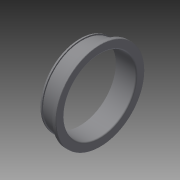
# Autodesk Inventor part: 32912_ir
Saved by Autodesk Inventor 2014 SP2 (Build 180246200, 246)
## iProperties
Created: 2018-11-12
Part Number: 32912_ir
Material: Generic
Catalog Web Link: www.cadenas.de
Description: BT1_001_101_ir-Tapered roller bearings, single row
Vendor: SKF
Document SubType Name: Modeling
Designer: psadmin
Manufacturer: SKF
Mass: 14.0656 g
Surface Area: 94.7996 cm^2
Volume: 14.0656 cm^3
Density: 1 g/cm^3
Appearance: PSOLRGB-175-175-175
Category: PARTsolutions
Company: SKF
Title: 32912_ir
Author: Cadenas PARTsolutions
Comments: Tapered roller bearings, single row
PSOL_IDENT_0: {$CADENAS_DATA\23d-libs\skf\bearings_units_and_housings\roller_bearings\tapered_roller_bearings\tape
PSOL_IDENT_1: red_roller_bearings_single_row\parts\bt1_001_101_ir.prj},166 {VTYP=3D},{NB=32912_ir},{LINA=32912_ir}
PSOL_IDENT_2: ,{NN=BT1_001_101_ir},{DATE=14.08.2018 07:35:10},{GEOMDATE=29.05.2018 10:14:25},{VERSION=},{LINEID=21
PSOL_IDENT_3: 40},{WBVAR=},{WBNUMERIC=}  {NB=32912_ir},{LINA=32912_ir},{KT=DUMMY},{DESIGNATION=32912},{DD=60.000},
PSOL_IDENT_4: {D=85.000},{T=17.000},{DD1=73.8000},{D1=MIN},{B=17.000},{C=14.000},{C1=MIN},{R12=1.0},{R34=1.0},{AA=
PSOL_IDENT_5: 15.45165},{PITCH=72.347},{DW=5.200},{LW=12.200},{RANGLE=1.600},{ALPHA=12.450},{DDAMAX=67},{DDAMIN=68
PSOL_IDENT_6: .0},{DAMIN=78},{DAMAX=78.0},{DBMIN=81},{CA=3},{CB=3.0},{RA=1.0},{RB=1.0},{LOAD1=53.200},{LOAD2=75.00
PSOL_IDENT_7: 0},{LOAD3=7.800},{SPEED1=6000},{SPEED2=7000},{EE=0.33},{Y=1.80},{Y0=1.0},{Y1=0},{X1=1},{X2=0.4},{X0=
PSOL_IDENT_8: 0.5},{Z=34},{II=1},{R1=0.00000231},{R2=10.9},{S1=0.009},{S2=2},{KZ=6},{KL=0.7},{BF=2},{MASS=0.302},{
PSOL_IDENT_9: PIM=PIM_BT1_001},{DESIGN=trb1},{HELP=0.000}
NN: BT1_001_101_ir
NT: Tapered roller bearings, single row
NB: 32912_ir
NBSYN: $DESIGNATION._ir
LINA: 32912_ir
DESIGNATION: 32912
DD: 60
D: 85
T: 17
DD1: 73.8
D1: 0
B: 17
C: 14
C1: 0
R12: 1
R34: 1
AA: 15.45165
PITCH: 72.347
DW: 5.2
LW: 12.2
RANGLE: 1.6
ALPHA: 12.45
DDAMAX: 67
DDAMIN: 68
DAMIN: 78
DAMAX: 78
DBMIN: 81
CA: 3
CB: 3
RA: 1
RB: 1
LOAD1: 53.2
LOAD2: 75
LOAD3: 7.8
SPEED1: 6000
SPEED2: 7000
EE: 0.33
Y: 1.8
Y0: 1
Y1: 0
X1: 1
X2: 0.4
X0: 0.5
Z: 34
II: 1
R1: 0.00000231
R2: 10.9
S1: 0.009
S2: 2
KZ: 6
KL: 0.7
BF: 2
MASS: 0.302
PIM: PIM_BT1_001
SUPPLIER: SKF
ARTICLENO: 32912_ir
BOMINFO: 32912_ir
CREATOR: CADENAS GmbH
Autodesk Inventor part; units mm, degrees
sketch "Sketch_1" plane through (0, 0, 0) normal (0, 0, 1) x (1, 0, 0)
  line L0 (16, 0) -> (0, 0)
  line L1 (0, 32.6773) -> (0, 30)
  line L2 (0, 30) -> (16, 30)
  arc A0 (16, 30) -> (17, 31) centre (16, 31) ccw
  line L3 (17, 31) -> (17, 36.65)
  line L4 (17, 36.65) -> (16.75, 36.9)
  line L5 (16.75, 36.9) -> (14.0638, 36.9)
  line L6 (14.0638, 36.9) -> (14.4927, 34.9577)
  line L7 (14.4927, 34.9577) -> (1.8039, 32.3617)
  line L8 (1.8039, 32.3617) -> (1.6171, 33.2081)
  line L9 (1.6171, 33.2081) -> (0.1959, 32.9174)
  line L10 (0.1959, 32.9174) -> (0, 32.6773)
  constraints: 22 end point, 2 point on circle, 1 centre point
revolve "Revolution1" add sketch "Sketch_1" angle 360 about axis through (16, 0, 0) along (1, 0, 0)
ref_plane "inner_ring_XY" through (0, 0, 0) normal (0, 0, 1) x (1, 0, 0)
ref_plane "inner_ring_YZ" through (0, 0, 0) normal (1, 0, 0) x (0, 1, 0)
ref_plane "inner_ring_ZX" through (0, 0, 0) normal (0, 1, 0) x (0, 0, 1)
body "Solid1"
